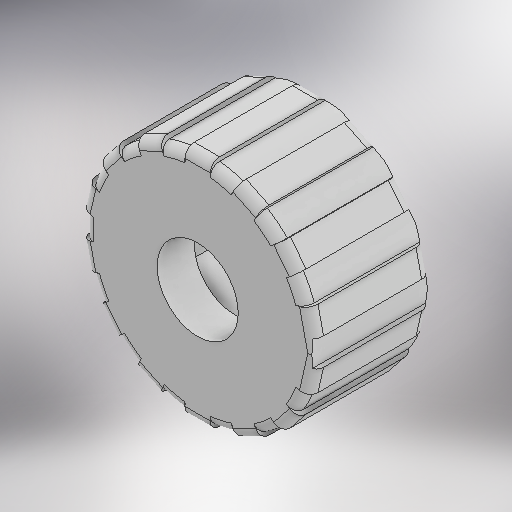
# Autodesk Inventor part: knob._375ipt
Saved by Autodesk Inventor 2026.2 (Build 302298000, 298)
## iProperties
Created: 2026-01-14
Part Number: knob._375ipt
Material: Generic
Document SubType Name: Modeling
Designer: bjones
Density: 1 g/cm^3
Appearance: Default
Author: bjones
Autodesk Inventor part; units mm, degrees
ref_plane "YZ Plane" through (0, 0, 0) normal (1, 0, 0) x (0, 1, 0)
ref_plane "XZ Plane" through (0, 0, 0) normal (0, 1, 0) x (-1, 0, 0)
ref_plane "XY Plane" through (0, 0, 0) normal (0, 0, 1) x (1, 0, 0)
sketch "Sketch1" plane through (0, 0, 0) normal (0, 0, 1) x (1, 0, 0)
  line L0 (0, 0) -> (0, 9.0967)
  line L1 (0, 0) -> (8.6249, 0)
  line L2 (0, 6.5258) -> (5.6515, 3.2629)
  line L3 (5.6515, 3.2629) -> (5.6515, -3.2629)
  line L4 (5.6515, -3.2629) -> (0, -6.5258)
  line L5 (0, -6.5258) -> (-5.6515, -3.2629)
  line L6 (-5.6515, -3.2629) -> (-5.6515, 3.2629)
  line L7 (-5.6515, 3.2629) -> (0, 6.5258)
  line L8 (-1.0357, 9.525) -> (1.0357, 9.525)
  line L9 (1.0357, 9.525) -> (1.0357, 6.7271)
  line L10 (1.0357, 6.7271) -> (-1.0357, 6.7271)
  line L11 (-1.0357, 6.7271) -> (-1.0357, 9.525)
  line L12 (-5.0659, 8.1324) -> (-3.1996, 9.0311)
  line L13 (-3.8519, 5.6115) -> (-5.0659, 8.1324)
  line L14 (-3.1996, 9.0311) -> (-1.9856, 6.5103)
  line L15 (-8.0927, 5.129) -> (-6.8012, 6.7485)
  line L16 (-5.9052, 3.3845) -> (-8.0927, 5.129)
  line L17 (-6.8012, 6.7485) -> (-4.6137, 5.004)
  line L18 (-9.5167, 1.1098) -> (-9.0557, 3.1293)
  line L19 (-6.7889, 0.4872) -> (-9.5167, 1.1098)
  line L20 (-9.0557, 3.1293) -> (-6.328, 2.5067)
  line L21 (-9.0557, -3.1293) -> (-9.5167, -1.1098)
  line L22 (-6.328, -2.5067) -> (-9.0557, -3.1293)
  line L23 (-9.5167, -1.1098) -> (-6.7889, -0.4872)
  line L24 (-6.8012, -6.7485) -> (-8.0927, -5.129)
  line L25 (-4.6137, -5.004) -> (-6.8012, -6.7485)
  line L26 (-8.0927, -5.129) -> (-5.9052, -3.3845)
  line L27 (-3.1996, -9.0311) -> (-5.0659, -8.1324)
  line L28 (-1.9856, -6.5103) -> (-3.1996, -9.0311)
  line L29 (-5.0659, -8.1324) -> (-3.8519, -5.6115)
  line L30 (1.0357, -9.525) -> (-1.0357, -9.525)
  line L31 (1.0357, -6.7271) -> (1.0357, -9.525)
  line L32 (-1.0357, -9.525) -> (-1.0357, -6.7271)
  line L33 (5.0659, -8.1324) -> (3.1996, -9.0311)
  line L34 (3.8519, -5.6115) -> (5.0659, -8.1324)
  line L35 (3.1996, -9.0311) -> (1.9856, -6.5103)
  line L36 (8.0927, -5.129) -> (6.8012, -6.7485)
  line L37 (5.9052, -3.3845) -> (8.0927, -5.129)
  line L38 (6.8012, -6.7485) -> (4.6137, -5.004)
  line L39 (9.5167, -1.1098) -> (9.0557, -3.1293)
  line L40 (6.7889, -0.4872) -> (9.5167, -1.1098)
  line L41 (9.0557, -3.1293) -> (6.328, -2.5067)
  line L42 (9.0557, 3.1293) -> (9.5167, 1.1098)
  line L43 (6.328, 2.5067) -> (9.0557, 3.1293)
  line L44 (9.5167, 1.1098) -> (6.7889, 0.4872)
  line L45 (6.8012, 6.7485) -> (8.0927, 5.129)
  line L46 (4.6137, 5.004) -> (6.8012, 6.7485)
  line L47 (8.0927, 5.129) -> (5.9052, 3.3845)
  line L48 (3.1996, 9.0311) -> (5.0659, 8.1324)
  line L49 (1.9856, 6.5103) -> (3.1996, 9.0311)
  line L50 (5.0659, 8.1324) -> (3.8519, 5.6115)
  circle A0 centre (0, 0) radius 9.271
  point P0 (1.0357, 9.213)
  point P1 (-1.0357, 9.213)
  point P2 (-3.0642, 8.75)
  point P3 (-4.9305, 7.8512)
  point P4 (-6.5572, 6.5539)
  point P5 (-7.8487, 4.9344)
  point P6 (-8.7515, 3.0598)
  point P7 (-9.2124, 1.0403)
  point P8 (-9.2124, -1.0403)
  point P9 (-8.7515, -3.0598)
  point P10 (-7.8487, -4.9344)
  point P11 (-6.5572, -6.5539)
  point P12 (-4.9305, -7.8512)
  point P13 (-3.0642, -8.75)
  point P14 (-1.0357, -9.213)
  point P15 (1.0357, -9.213)
  point P16 (3.0642, -8.75)
  point P17 (4.9305, -7.8512)
  point P18 (6.5572, -6.5539)
  point P19 (7.8487, -4.9344)
  point P20 (8.7515, -3.0598)
  point P21 (9.2124, -1.0403)
  point P22 (9.2124, 1.0403)
  point P23 (8.7515, 3.0598)
  point P24 (7.8487, 4.9344)
  point P25 (6.5572, 6.5539)
  point P26 (4.9305, 7.8512)
  point P27 (3.0642, 8.75)
  dimension "d6" = 18.542
  dimension "d0" = 11.303
  dimension "d4" = 360
  constraints: 102 end point, 2 coincident, 2 horizontal, 2 parallel, 1 perpendicular, 1 vertical, 115 other
  measures "d0" distance between parallel lines of L5 L2
extrude "Extrusion1" add sketch "Sketch1" along normal blind 9.525
sketch "Sketch2" plane through (0, 0, 9.525) normal (0, 0, 1) x (1, 0, 0)
  line L0 (1.0357, 9.525) -> (-1.0357, 9.525) projected
  line L1 (-1.0357, 9.525) -> (-1.0357, 9.213) projected
  arc A0 (-1.0357, 9.213) -> (-3.0642, 8.75) centre (0, 0) ccw projected
  line L2 (-3.0642, 8.75) -> (-3.1996, 9.0311) projected
  line L3 (-3.1996, 9.0311) -> (-5.0659, 8.1324) projected
  line L4 (-5.0659, 8.1324) -> (-4.9305, 7.8512) projected
  arc A1 (-4.9305, 7.8512) -> (-6.5572, 6.5539) centre (0, 0) ccw projected
  line L5 (-6.5572, 6.5539) -> (-6.8012, 6.7485) projected
  line L6 (-6.8012, 6.7485) -> (-8.0927, 5.129) projected
  line L7 (-8.0927, 5.129) -> (-7.8487, 4.9344) projected
  arc A2 (-7.8487, 4.9344) -> (-8.7515, 3.0598) centre (0, 0) ccw projected
  line L8 (-8.7515, 3.0598) -> (-9.0557, 3.1293) projected
  line L9 (-9.0557, 3.1293) -> (-9.5167, 1.1098) projected
  line L10 (-9.5167, 1.1098) -> (-9.2124, 1.0403) projected
  arc A3 (-9.2124, 1.0403) -> (-9.2124, -1.0403) centre (0, 0) ccw projected
  line L11 (-9.2124, -1.0403) -> (-9.5167, -1.1098) projected
  line L12 (-9.5167, -1.1098) -> (-9.0557, -3.1293) projected
  line L13 (-9.0557, -3.1293) -> (-8.7515, -3.0598) projected
  arc A4 (-8.7515, -3.0598) -> (-7.8487, -4.9344) centre (0, 0) ccw projected
  line L14 (-7.8487, -4.9344) -> (-8.0927, -5.129) projected
  line L15 (-8.0927, -5.129) -> (-6.8012, -6.7485) projected
  line L16 (-6.8012, -6.7485) -> (-6.5572, -6.5539) projected
  arc A5 (-6.5572, -6.5539) -> (-4.9305, -7.8512) centre (0, 0) ccw projected
  line L17 (-4.9305, -7.8512) -> (-5.0659, -8.1324) projected
  line L18 (-5.0659, -8.1324) -> (-3.1996, -9.0311) projected
  line L19 (-3.1996, -9.0311) -> (-3.0642, -8.75) projected
  arc A6 (-3.0642, -8.75) -> (-1.0357, -9.213) centre (0, 0) ccw projected
  line L20 (-1.0357, -9.213) -> (-1.0357, -9.525) projected
  line L21 (-1.0357, -9.525) -> (1.0357, -9.525) projected
  line L22 (1.0357, -9.525) -> (1.0357, -9.213) projected
  arc A7 (1.0357, -9.213) -> (3.0642, -8.75) centre (0, 0) ccw projected
  line L23 (3.0642, -8.75) -> (3.1996, -9.0311) projected
  line L24 (3.1996, -9.0311) -> (5.0659, -8.1324) projected
  line L25 (5.0659, -8.1324) -> (4.9305, -7.8512) projected
  arc A8 (4.9305, -7.8512) -> (6.5572, -6.5539) centre (0, 0) ccw projected
  line L26 (6.5572, -6.5539) -> (6.8012, -6.7485) projected
  line L27 (6.8012, -6.7485) -> (8.0927, -5.129) projected
  line L28 (8.0927, -5.129) -> (7.8487, -4.9344) projected
  arc A9 (7.8487, -4.9344) -> (8.7515, -3.0598) centre (0, 0) ccw projected
  line L29 (8.7515, -3.0598) -> (9.0557, -3.1293) projected
  line L30 (9.0557, -3.1293) -> (9.5167, -1.1098) projected
  line L31 (9.5167, -1.1098) -> (9.2124, -1.0403) projected
  arc A10 (9.2124, -1.0403) -> (9.2124, 1.0403) centre (0, 0) ccw projected
  line L32 (9.2124, 1.0403) -> (9.5167, 1.1098) projected
  line L33 (9.5167, 1.1098) -> (9.0557, 3.1293) projected
  line L34 (9.0557, 3.1293) -> (8.7515, 3.0598) projected
  arc A11 (8.7515, 3.0598) -> (7.8487, 4.9344) centre (0, 0) ccw projected
  line L35 (7.8487, 4.9344) -> (8.0927, 5.129) projected
  line L36 (8.0927, 5.129) -> (6.8012, 6.7485) projected
  line L37 (6.8012, 6.7485) -> (6.5572, 6.5539) projected
  arc A12 (6.5572, 6.5539) -> (4.9305, 7.8512) centre (0, 0) ccw projected
  line L38 (4.9305, 7.8512) -> (5.0659, 8.1324) projected
  line L39 (5.0659, 8.1324) -> (3.1996, 9.0311) projected
  line L40 (3.1996, 9.0311) -> (3.0642, 8.75) projected
  arc A13 (3.0642, 8.75) -> (1.0357, 9.213) centre (0, 0) ccw projected
  line L41 (1.0357, 9.213) -> (1.0357, 9.525) projected
  line L42 (0, 6.5258) -> (5.6515, 3.2629) projected
  line L43 (5.6515, 3.2629) -> (5.6515, -3.2629) projected
  line L44 (5.6515, -3.2629) -> (0, -6.5258) projected
  line L45 (0, -6.5258) -> (-5.6515, -3.2629) projected
  line L46 (-5.6515, -3.2629) -> (-5.6515, 3.2629) projected
  line L47 (-5.6515, 3.2629) -> (0, 6.5258) projected
  circle A14 centre (0, 0) radius 3.302
  dimension "d11" = 6.604
  constraints: 1 centre point, 1 coincident
  measures "d11" diameter of A14
extrude "Extrusion2" add sketch "Sketch2" against normal blind 3.048 contours L42 L43 L44 L45 L46 L47
sketch "Sketch3" plane through (0, 0, 0) normal (0, 0, -1) x (-1, 0, 0)
  line L0 (-1.0357, 9.525) -> (1.0357, 9.525) projected
  line L1 (-1.0357, 9.213) -> (-1.0357, 9.525) projected
  arc A0 (-1.0357, 9.213) -> (-3.0642, 8.75) centre (0, 0) ccw projected
  line L2 (-3.1996, 9.0311) -> (-3.0642, 8.75) projected
  line L3 (-5.0659, 8.1324) -> (-3.1996, 9.0311) projected
  line L4 (-4.9305, 7.8512) -> (-5.0659, 8.1324) projected
  arc A1 (-4.9305, 7.8512) -> (-6.5572, 6.5539) centre (0, 0) ccw projected
  line L5 (-6.8012, 6.7485) -> (-6.5572, 6.5539) projected
  line L6 (-8.0927, 5.129) -> (-6.8012, 6.7485) projected
  line L7 (-7.8487, 4.9344) -> (-8.0927, 5.129) projected
  arc A2 (-7.8487, 4.9344) -> (-8.7515, 3.0598) centre (0, 0) ccw projected
  line L8 (-9.0557, 3.1293) -> (-8.7515, 3.0598) projected
  line L9 (-9.5167, 1.1098) -> (-9.0557, 3.1293) projected
  line L10 (-9.2124, 1.0403) -> (-9.5167, 1.1098) projected
  arc A3 (-9.2124, 1.0403) -> (-9.2124, -1.0403) centre (0, 0) ccw projected
  line L11 (-9.5167, -1.1098) -> (-9.2124, -1.0403) projected
  line L12 (-9.0557, -3.1293) -> (-9.5167, -1.1098) projected
  line L13 (-8.7515, -3.0598) -> (-9.0557, -3.1293) projected
  arc A4 (-8.7515, -3.0598) -> (-7.8487, -4.9344) centre (0, 0) ccw projected
  line L14 (-8.0927, -5.129) -> (-7.8487, -4.9344) projected
  line L15 (-6.8012, -6.7485) -> (-8.0927, -5.129) projected
  line L16 (-6.5572, -6.5539) -> (-6.8012, -6.7485) projected
  arc A5 (-6.5572, -6.5539) -> (-4.9305, -7.8512) centre (0, 0) ccw projected
  line L17 (-5.0659, -8.1324) -> (-4.9305, -7.8512) projected
  line L18 (-3.1996, -9.0311) -> (-5.0659, -8.1324) projected
  line L19 (-3.0642, -8.75) -> (-3.1996, -9.0311) projected
  arc A6 (-3.0642, -8.75) -> (-1.0357, -9.213) centre (0, 0) ccw projected
  line L20 (-1.0357, -9.525) -> (-1.0357, -9.213) projected
  line L21 (1.0357, -9.525) -> (-1.0357, -9.525) projected
  line L22 (1.0357, -9.213) -> (1.0357, -9.525) projected
  arc A7 (1.0357, -9.213) -> (3.0642, -8.75) centre (0, 0) ccw projected
  line L23 (3.1996, -9.0311) -> (3.0642, -8.75) projected
  line L24 (5.0659, -8.1324) -> (3.1996, -9.0311) projected
  line L25 (4.9305, -7.8512) -> (5.0659, -8.1324) projected
  arc A8 (4.9305, -7.8512) -> (6.5572, -6.5539) centre (0, 0) ccw projected
  line L26 (6.8012, -6.7485) -> (6.5572, -6.5539) projected
  line L27 (8.0927, -5.129) -> (6.8012, -6.7485) projected
  line L28 (7.8487, -4.9344) -> (8.0927, -5.129) projected
  arc A9 (7.8487, -4.9344) -> (8.7515, -3.0598) centre (0, 0) ccw projected
  line L29 (9.0557, -3.1293) -> (8.7515, -3.0598) projected
  line L30 (9.5167, -1.1098) -> (9.0557, -3.1293) projected
  line L31 (9.2124, -1.0403) -> (9.5167, -1.1098) projected
  arc A10 (9.2124, -1.0403) -> (9.2124, 1.0403) centre (0, 0) ccw projected
  line L32 (9.5167, 1.1098) -> (9.2124, 1.0403) projected
  line L33 (9.0557, 3.1293) -> (9.5167, 1.1098) projected
  line L34 (8.7515, 3.0598) -> (9.0557, 3.1293) projected
  arc A11 (8.7515, 3.0598) -> (7.8487, 4.9344) centre (0, 0) ccw projected
  line L35 (8.0927, 5.129) -> (7.8487, 4.9344) projected
  line L36 (6.8012, 6.7485) -> (8.0927, 5.129) projected
  line L37 (6.5572, 6.5539) -> (6.8012, 6.7485) projected
  arc A12 (6.5572, 6.5539) -> (4.9305, 7.8512) centre (0, 0) ccw projected
  line L38 (5.0659, 8.1324) -> (4.9305, 7.8512) projected
  line L39 (3.1996, 9.0311) -> (5.0659, 8.1324) projected
  line L40 (3.0642, 8.75) -> (3.1996, 9.0311) projected
  arc A13 (3.0642, 8.75) -> (1.0357, 9.213) centre (0, 0) ccw projected
  line L41 (1.0357, 9.525) -> (1.0357, 9.213) projected
  line L42 (0, 6.5258) -> (-5.6515, 3.2629) projected
  line L43 (5.6515, 3.2629) -> (0, 6.5258) projected
  line L44 (5.6515, -3.2629) -> (5.6515, 3.2629) projected
  line L45 (0, -6.5258) -> (5.6515, -3.2629) projected
  line L46 (-5.6515, -3.2629) -> (0, -6.5258) projected
  line L47 (-5.6515, 3.2629) -> (-5.6515, -3.2629) projected
  circle A14 centre (0, 0) radius 7.9375
  dimension "d12" = 15.875
  constraints: 1 centre point, 1 coincident
  measures "d12" diameter of A14
extrude "Extrusion3" cut sketch "Sketch3" against normal blind 2.54 contours A14
fillet "Fillet1" radius 0.762 44 edges at (7.9375, 0, 0) (7.9375, 0, 2.54) (0, 9.525, 9.525) (-4.1327, 8.5817, 9.525) (-7.4469, 5.9387, 9.525) (-9.2862, 2.1195, 9.525) (-9.2862, -2.1195, 9.525) (-7.4469, -5.9387, 9.525) (-4.1327, -8.5817, 9.525) (0, -9.525, 9.525) (4.1327, -8.5817, 9.525) (7.4469, -5.9387, 9.525) (9.2862, -2.1195, 9.525) (9.2862, 2.1195, 9.525) (8.3529, 4.0225, 9.525) (5.7804, 7.2484, 9.525) (2.063, 9.0386, 9.525) (-2.063, 9.0386, 9.525) (-5.7804, 7.2484, 9.525) (-8.3529, 4.0225, 9.525) (-9.271, 0, 9.525) (-8.3529, -4.0225, 9.525) (-5.7804, -7.2484, 9.525) (-2.063, -9.0386, 9.525) (2.063, -9.0386, 9.525) (5.7804, -7.2484, 9.525) (8.3529, -4.0225, 9.525) (5.6515, -3.2629, 4.5085) (7.4469, 5.9387, 9.525) (4.1327, 8.5817, 9.525) (-4.1327, 8.5817, 0) (0, 9.525, 0) (4.1327, 8.5817, 0) (7.4469, 5.9387, 0) (9.2862, 2.1195, 0) (9.2862, -2.1195, 0) (7.4469, -5.9387, 0) (4.1327, -8.5817, 0) (0, -9.525, 0) (-4.1327, -8.5817, 0) (-7.4469, -5.9387, 0) (-9.2862, -2.1195, 0) (-9.2862, 2.1195, 0) (-7.4469, 5.9387, 0)
body "Solid1"
